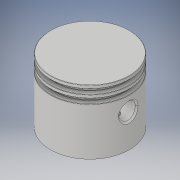
# Autodesk Inventor part: Component 11 (Piston)
Saved by Autodesk Inventor 2018 (Build 220112000, 112)
## iProperties
Created: 2023-03-14
Part Number: Component 11 (Piston)
Material: Generic
Document SubType Name: Modeling
Designer: Habib Mohamed
Density: 1 g/cm^3
Appearance: Default
Author: Habib Mohamed
Autodesk Inventor part; units mm, degrees
ref_plane "YZ Plane" through (0, 0, 0) normal (1, 0, 0) x (0, 1, 0)
ref_plane "XZ Plane" through (0, 0, 0) normal (0, 1, 0) x (-1, 0, 0)
ref_plane "XY Plane" through (0, 0, 0) normal (0, 0, 1) x (1, 0, 0)
sketch "Sketch1" plane through (0, 0, 0) normal (1, 0, 0) x (0, 1, 0)
  line L0 (0, 0) -> (19.5, 0) construction
  line L1 (19.5, 0) -> (19.5, 11.9)
  line L2 (19.4, 12) -> (18.6, 12)
  line L3 (18.5, 11.9) -> (18.5, 10.6)
  line L4 (18.4, 10.5) -> (17.1, 10.5)
  line L5 (17, 10.6) -> (17, 11.9)
  line L6 (16.9, 12) -> (16.1, 12)
  line L7 (16, 11.9) -> (16, 10.6)
  line L8 (15.9, 10.5) -> (14.6, 10.5)
  line L9 (14.5, 10.6) -> (14.5, 11.9)
  line L10 (14.4, 12) -> (0, 12)
  line L11 (0, 12) -> (0, 11)
  line L12 (0, 11) -> (4, 11)
  line L13 (5, 10) -> (5, 0)
  arc A0 (5, 10) -> (4, 11) centre (4, 10) ccw
  arc A1 (19.5, 11.9) -> (19.4, 12) centre (19.4, 11.9) ccw
  arc A2 (18.6, 12) -> (18.5, 11.9) centre (18.6, 11.9) ccw
  arc A3 (17, 11.9) -> (16.9, 12) centre (16.9, 11.9) ccw
  arc A4 (16.1, 12) -> (16, 11.9) centre (16.1, 11.9) ccw
  line L14 (0, 0) -> (0, 16.1178) construction
  arc A5 (18.4, 10.5) -> (18.5, 10.6) centre (18.4, 10.6) ccw
  arc A6 (17, 10.6) -> (17.1, 10.5) centre (17.1, 10.6) ccw
  arc A7 (15.9, 10.5) -> (16, 10.6) centre (15.9, 10.6) ccw
  arc A8 (14.5, 10.6) -> (14.6, 10.5) centre (14.6, 10.6) ccw
  arc A9 (14.5, 11.9) -> (14.4, 12) centre (14.4, 11.9) ccw
  line L15 (19.5, 0) -> (5, 0)
  point P0 (19.5, 12)
  point P1 (18.5, 12)
  point P2 (18.5, 10.5)
  point P3 (17, 10.5)
  point P4 (17, 12)
  point P5 (16, 12)
  point P6 (16, 10.5)
  point P7 (14.5, 10.5)
  point P8 (14.5, 12)
  dimension "d0" = 12
  dimension "d3" = 1
  dimension "d4" = 1.5
  dimension "d5" = 1
  dimension "d6" = 1.5
  dimension "d7" = 5
  dimension "d8" = 1
  dimension "d9" = 0.1
  dimension "d10" = 19.5
  dimension "d11" = 0.1
  constraints: 32 end point, 25 point on line, 20 point on circle, 20 tangent, 10 centre point, 9 perpendicular, 7 equal radius, 4 collinear, 2 vertical, 1 horizontal
  measures "d0" distance of L0.end point (19.5, 12)
  measures "d3" distance of point (19.5, 12) point (18.5, 12)
  measures "d4" distance of point (18.5, 10.5) point (17, 10.5)
  measures "d5" distance of L10.end L11.end
  measures "d6" distance of point (18.5, 12) point (18.5, 10.5)
  measures "d7" distance between parallel lines of L13 L11
  measures "d8" radius of A0
  measures "d9" radius of A1
  measures "d10" distance between parallel lines of L1 L14
  measures "d11" radius of A5
revolve "Revolution1" add sketch "Sketch1" angle 360 about axis through (0, 19.5, 0) along (0, -1, 0)
sketch "Sketch2" plane through (0, 5, 0) normal (0, -1, 0) x (1, 0, 0)
  line L0 (0, 5) -> (0, -5) construction
  line L1 (-5, 5) -> (-5, -5)
  line L2 (5, -5) -> (5, 5)
  arc A0 (5, 5) -> (-5, 5) centre (0, 5) ccw
  arc A1 (-5, -5) -> (5, -5) centre (0, -5) ccw
  point P0 (0, 0)
  dimension "d13" = 10
  dimension "d14" = 5
  constraints: 8 end point, 4 point on circle, 4 tangent, 2 centre point, 1 midpoint, 1 parallel, 1 vertical
  measures "d13" distance of L0.start L0.end
  measures "d14" radius of A1
extrude "Extrusion1" cut sketch "Sketch2" against normal blind 11
sketch "Sketch3" plane through (0, 0, 0) normal (1, 0, 0) x (0, 1, 0)
  circle A0 centre (10, 0) radius 2.5
  line L0 (0, 0) -> (23.6233, 0) construction
  dimension "d17" = 5
  dimension "d18" = 10
  constraints: 2 end point, 1 centre point, 1 horizontal, 1 point on line
  measures "d17" diameter of A0
  measures "d18" distance of L0.start A0.centre
extrude "Extrusion2" cut sketch "Sketch3" along normal mid plane 36.75
chamfer "Chamfer1" distance 0.5 angle 45 4 edges at (11.9595, 7.7023, 0.9853) (-11.9595, 7.7023, 0.9853) (-5, 7.5, 0) (5, 7.5, 0)
sketch "Sketch4" plane through (0, 5, 0) normal (0, -1, 0) x (1, 0, 0)
  point P0 (0, 0)
  point P1 (8, 0)
  point P2 (-8, 0)
  dimension "d24" = 8
  dimension "d25" = 8
  constraints: 2 horizontal alignment
  measures "d24" distance of point (0, 0) point (8, 0)
  measures "d25" distance of point (-8, 0) point (0, 0)
hole "Hole1" at (8, 5, 0) at (-8, 5, 0) direction (0, 1, 0) diameter 2.013 end up to face face through (0, 10, 0) facing (1, 0, 0) round with radius 2.5 far side no thread size "M2.5x0.45" class "6H" standard "ANSI Metric M Profile"
fillet "Fillet1" radius 1 4 edges at (5, 16, 0) (0, 16, -10) (-5, 16, 0) (0, 16, 10)
equation "\"d25\" = d24"
body "Solid1"
